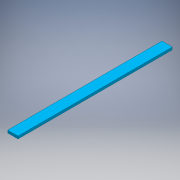
# Autodesk Inventor part: Pieza Prueba Small
Saved by Autodesk Inventor 2018.3 (Build 223284000, 284)
## iProperties
Created: 2019-05-20
Part Number: Pieza Prueba Small
Material: Generic
Document SubType Name: Modeling
Designer: Ivan
Density: 1 g/cm^3
Appearance: Default
Mass: 5.76 g
Surface Area: 39.36 cm^2
Volume: 5.76 cm^3
Author: Ivan
Autodesk Inventor part; units mm, degrees
ref_plane "YZ Plane" through (0, 0, 0) normal (1, 0, 0) x (0, 1, 0)
ref_plane "XZ Plane" through (0, 0, 0) normal (0, 1, 0) x (-1, 0, 0)
ref_plane "XY Plane" through (0, 0, 0) normal (0, 0, 1) x (1, 0, 0)
sketch "Sketch1" plane through (0, 0, 0) normal (0, 0, 1) x (1, 0, 0)
  line L0 (-4, 60) -> (4, 60)
  line L1 (4, 60) -> (4, -60)
  line L2 (4, -60) -> (-4, -60)
  line L3 (-4, -60) -> (-4, 60)
  point P0 (0, 0)
  point P1 (0, 60)
  point P2 (4, 0)
  dimension "d0" = 120
  dimension "d1" = 8
  constraints: 8 end point, 2 midpoint, 2 parallel, 1 horizontal, 1 horizontal alignment, 1 perpendicular, 1 vertical alignment
  measures "d0" distance of L0.end L1.end
  measures "d1" distance between parallel lines of L3 L1
extrude "Extrusion1" add sketch "Sketch1" along normal blind 2
body "Solid1"
